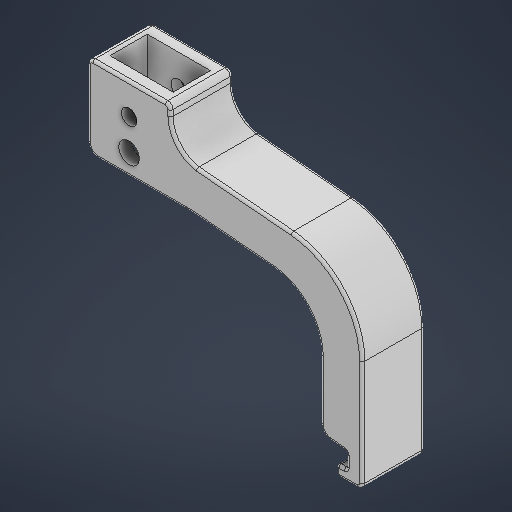
# Autodesk Inventor part: claw
Saved by Autodesk Inventor 2026.3 (Build 303398000, 398)
## iProperties
Created: 2026-06-24
Part Number: claw
Material: Generic
Document SubType Name: Modeling
Designer: frede
Density: 1 g/cm^3
Appearance: Default
Author: frede
Autodesk Inventor part; units mm, degrees
ref_plane "YZ Plane" through (0, 0, 0) normal (1, 0, 0) x (0, 1, 0)
ref_plane "XZ Plane" through (0, 0, 0) normal (0, 1, 0) x (-1, 0, 0)
ref_plane "XY Plane" through (0, 0, 0) normal (0, 0, 1) x (1, 0, 0)
sketch "Sketch1" plane through (0, 0, 0) normal (0, 0, 1) x (1, 0, 0)
  line L0 (0.5, -22.3753) -> (1.5, -22.3753)
  line L1 (2, -21.8753) -> (2, -19.8335)
  line L2 (0, -22.8753) -> (0, -23.8753)
  line L3 (0.5, -24.3753) -> (4, -24.3753)
  line L4 (5, -23.3753) -> (5, -2.9769)
  line L5 (-28.8732, 5.6247) -> (-46, 5.6247)
  circle A0 centre (-40, 9.6247) radius 2
  circle A1 centre (-40, 15.6247) radius 1.5
  line L6 (-48, 7.6247) -> (-48, 20.6247)
  line L7 (-40, 15.6247) -> (-40, 9.6247)
  line L8 (-32, 19.4876) -> (-32, 20.6247)
  line L9 (-33, 21.6247) -> (-47, 21.6247)
  arc A2 (-32, 19.4876) -> (-26.951, 13.5634) centre (-26, 19.4876) ccw
  arc A3 (-48, 7.6247) -> (-46, 5.6247) centre (-46, 7.6247) ccw
  arc A4 (-47, 21.6247) -> (-48, 20.6247) centre (-47, 20.6247) ccw
  arc A5 (-32, 20.6247) -> (-33, 21.6247) centre (-33, 20.6247) ccw
  arc A6 (5, -2.9769) -> (-8.6927, 11.966) centre (-10, -2.9769) ccw
  arc A7 (4, -24.3753) -> (5, -23.3753) centre (4, -23.3753) ccw
  arc A8 (0, -23.8753) -> (0.5, -24.3753) centre (0.5, -23.8753) ccw
  arc A9 (0.5, -22.3753) -> (0, -22.8753) centre (0.5, -22.8753) ccw
  arc A10 (1.5, -22.3753) -> (2, -21.8753) centre (1.5, -21.8753) ccw
  line L10 (-27.1301, 5.5486) -> (-12.1284, 4.2361)
  line L11 (-28, 5.6247) -> (-4.1886, 5.6247) construction
  line L12 (-26.951, 13.5634) -> (-8.6927, 11.966)
  line L13 (1.5436, -19.3354) -> (-1.1743, -19.0976)
  line L14 (2, -19.3753) -> (4.7283, -19.3753) construction
  line L15 (-3, -17.1052) -> (-3, -5.7259)
  arc A11 (-3, -5.7259) -> (-12.1284, 4.2361) centre (-13, -5.7259) ccw
  arc A12 (-27.1301, 5.5486) -> (-28.8732, 5.6247) centre (-28.8732, -14.3753) ccw
  arc A13 (-3, -17.1052) -> (-1.1743, -19.0976) centre (-1, -17.1052) ccw
  arc A14 (2, -19.8335) -> (1.5436, -19.3354) centre (1.5, -19.8335) ccw
  point P0 (2, -22.3753)
  point P1 (0, -24.3753)
  point P2 (5, -24.3753)
  point P3 (-48, 5.6247)
  point P4 (-3, -18.9379)
  point P5 (-3, 3.4374)
  dimension "d0" = 3
  dimension "d2" = 5
  dimension "d6" = 4
  dimension "d7" = 3
  dimension "d8" = 8
  dimension "d9" = 4
  dimension "d10" = 6
  dimension "d11" = 16
  dimension "d12" = 16
  dimension "d13" = 6
  dimension "d14" = 2
  dimension "d15" = 1
  dimension "d16" = 0.5
  dimension "d19" = 3
  dimension "d22" = 42
  dimension "d30" = 30
  dimension "d31" = 2
  dimension "d33" = 5
  dimension "d34" = 30
  dimension "d35" = 175
  dimension "d36" = 5
  dimension "d37" = 10
  dimension "d38" = 20
  dimension "d39" = 2
  dimension "d40" = 0.5
  dimension "d42" = 15
  dimension "d43" = 8
  constraints: 32 end point, 26 point on circle, 25 tangent, 16 point on line, 15 centre point, 6 vertical, 4 horizontal, 3 perpendicular, 2 equal radius, 1 equal length, 1 parallel
  measures "d0" distance of L14.start point (2, -22.375)
  measures "d2" distance of point (0, -24.375) point (5, -24.375)
  measures "d6" diameter of A0
  measures "d7" diameter of A1
  measures "d8" distance from line of point (-48, 5.625) L7
  measures "d9" distance from line of L5 L7.end
  measures "d10" distance of L7.start L7.end
  measures "d11" distance between parallel lines of L6 L8
  measures "d12" distance between parallel lines of L5 L9
  measures "d13" radius of A2
  measures "d14" radius of A3
  measures "d15" radius of A4
  measures "d16" radius of A8
  measures "d19" distance between parallel lines of L4 L1
  measures "d22" distance between parallel lines of L1 L7
  measures "d30" distance between parallel lines of L3 L5
  measures "d31" distance between parallel lines of L3 L0
  measures "d33" angle of L10 L11
  measures "d34" distance from line of L1 L11.start
  measures "d35" angle of L14 L13
  measures "d36" distance from line of L1 point (-3, -18.938)
  measures "d37" radius of A11
  measures "d38" radius of A12
  measures "d39" radius of A13
  measures "d40" radius of A14
  measures "d42" radius of A6
  measures "d43" distance between parallel lines of L10 L12
extrude "Extrusion1" add sketch "Sketch1" along normal blind 12
fillet "Fillet1" radius 0.5 2 edges at (-42, 9.6247, 0) (-41.5, 15.6247, 0)
fillet "Fillet2" radius 0.5 36 edges at (-32, 20.0561, 12) (-32.2929, 21.3318, 12) (-40, 21.6247, 12) (1.0592, 7.157, 12) (5, -13.1761, 12) (4.7071, -24.0824, 12) (2.25, -24.3753, 12) (0.1464, -24.2289, 12) (0, -23.3753, 12) (0.1464, -22.5218, 12) (1, -22.3753, 12) (1.8536, -22.2289, 12) (2, -20.8544, 12) (-30.5665, 15.5957, 12) (-32, 20.0561, 0) (-32.2929, 21.3318, 0) (-40, 21.6247, 0) (-47.7071, 21.3318, 0) (-48, 14.1247, 0) (-47.4142, 6.2104, 0) (-37.4366, 5.6247, 0) (1.0592, 7.157, 0) (5, -13.1761, 0) (4.7071, -24.0824, 0) (2.25, -24.3753, 0) (0.1464, -24.2289, 0) (0, -23.3753, 0) (0.1464, -22.5218, 0) (1, -22.3753, 0) (1.8536, -22.2289, 0) (2, -20.8544, 0) (-30.5665, 15.5957, 0) (-37.4366, 5.6247, 12) (-48, 14.1247, 12) (-47.7071, 21.3318, 12) (-47.4142, 6.2104, 12)
sketch "Sketch3" plane through (-47, 21.6247, 0.5) normal (0, 1, 0) x (1, 0, 0)
  line L0 (0.9, -1.9) -> (13.1, -1.9)
  line L1 (13.1, -1.9) -> (13.1, -9.1)
  line L2 (13.1, -9.1) -> (0.9, -9.1)
  line L3 (0.9, -9.1) -> (0.9, -1.9)
  line L4 (15, 0) -> (15, -11) projected
  line L5 (-1, 0) -> (-1, -11) projected
  line L6 (0, -11.5) -> (14, -11.5) projected
  line L7 (14, 0.5) -> (0, 0.5) projected
  point P0 (47, 0.5)
  dimension "d44" = 12.2
  dimension "d45" = 7.2
  dimension "d46" = 16
  dimension "d47" = 12
  dimension "d48" = 2.4
  dimension "d49" = 1.9
  constraints: 8 end point, 2 parallel, 1 horizontal, 1 perpendicular
  measures "d44" distance of L1.end L2.end
  measures "d45" distance of L0.end L1.end
  measures "d46" distance between parallel lines of L4 L5
  measures "d47" distance between parallel lines of L6 L7
  measures "d48" distance between parallel lines of L7 L0
  measures "d49" distance between parallel lines of L5 L3
extrude "Extrusion3" cut sketch "Sketch3" against normal up to surface (16 mm away)
equation "\"d8\" = 0.5 * d11"
equation "\"d48\" = -0.5 * d45 + 0.5 * d47"
equation "\"d49\" = -0.5 * d44 + 0.5 * d46"
body "Solid1"
